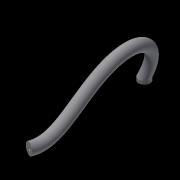
# Autodesk Inventor part: 3d_LM - Tubo 1x1-2
Saved by Autodesk Inventor 2018 (Build 220112000, 112)
## iProperties
Created: 2025-09-03
Part Number: 3d_LM - Tubo 1x1-2
Material: Genérico
Document SubType Name: Modeling
Designer: mbs18
Density: 1 g/cm^3
Appearance: Valor por defecto
Author: mbs18
Autodesk Inventor part; units mm, degrees
ref_plane "YZ Plane" through (0, 0, 0) normal (1, 0, 0) x (0, 1, 0)
ref_plane "XZ Plane" through (0, 0, 0) normal (0, 1, 0) x (-1, 0, 0)
ref_plane "XY Plane" through (0, 0, 0) normal (0, 0, 1) x (1, 0, 0)
sketch "Sketch1" plane through (0, 0, 0) normal (0, 0, 1) x (1, 0, 0)
  circle A0 centre (0, 0) radius 1.75
  circle A1 centre (0, 0) radius 0.5
  dimension "d0" = 3.5
  dimension "d1" = 1
  constraints: 2 centre point, 2 coincident
  measures "d0" diameter of A0
  measures "d1" diameter of A1
extrude "Extrusion1" add sketch "Sketch1" along normal blind 1
sketch "Sketch9" plane through (0, 0, 1) normal (0, 0, 1) x (1, 0, 0)
  circle A0 centre (0, 0) radius 0.5 projected
  circle A1 centre (0, 0) radius 1.75 projected
sketch3d "3D Sketch8"
  spline S0 degree 4 poles (0, 0, 1) (5.1319, 5.755, 17.5754) (1.3737, -19.5029, 21.3345) (4.4744, -23.8794, -0.7581) (4.1505, -39.5714, 3.5818) knots 0 0 0 0 0 1 1 1 1 1
sweep "Sweep9" add profiles "Sketch9" path "3D Sketch8"
body "Solid1"
